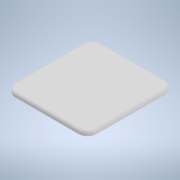
# Autodesk Inventor part: micro lipo lid
Saved by Autodesk Inventor 2020 (Build 240168000, 168)
## iProperties
Created: 2020-08-31
Part Number: micro lipo lid
Material: Generic
Document SubType Name: Modeling
Designer: mulve
Density: 1 g/cm^3
Appearance: Default
Author: mulve
Autodesk Inventor part; units mm, degrees
ref_plane "YZ Plane" through (0, 0, 0) normal (1, 0, 0) x (0, 1, 0)
ref_plane "XZ Plane" through (0, 0, 0) normal (0, 1, 0) x (-1, 0, 0)
ref_plane "XY Plane" through (0, 0, 0) normal (0, 0, 1) x (1, 0, 0)
sketch "Sketch1" plane through (0, 0, 0) normal (0, 1, 0) x (-1, 0, 0)
  line L0 (0, 0) -> (22.86, 0)
  line L1 (22.86, 0) -> (22.86, -24.13)
  line L2 (22.86, -24.13) -> (0, -24.13)
  line L3 (0, -24.13) -> (0, 0)
  dimension "d0" = 24.13
  dimension "d1" = 22.86
  constraints: 8 end point, 2 parallel, 1 horizontal, 1 perpendicular
  measures "d0" distance of L0.end L1.end
  measures "d1" distance of L1.end L2.end
extrude "Extrusion1" add sketch "Sketch1" along normal blind 2
sketch "Sketch2" plane through (0, 0, 0) normal (0, -1, 0) x (1, 0, 0)
  line L0 (-1.27, -1.27) -> (-21.59, -1.27)
  line L1 (-21.59, -1.27) -> (-21.59, -22.86)
  line L2 (-21.59, -22.86) -> (-1.27, -22.86)
  line L3 (-1.27, -22.86) -> (-1.27, -1.27)
  line L4 (-22.86, 0) -> (0, 0) projected
  line L5 (0, -24.13) -> (-22.86, -24.13) projected
  line L6 (0, 0) -> (0, -24.13) projected
  line L7 (-22.86, -24.13) -> (-22.86, 0) projected
  line L8 (0, 0) -> (0, -24.13) projected
  line L9 (0, 0) -> (-22.86, 0)
  line L10 (-22.86, 0) -> (-22.86, -24.13)
  line L11 (-22.86, -24.13) -> (0, -24.13)
  line L12 (0, -24.13) -> (0, 0)
  dimension "d4" = 20.32
  dimension "d5" = 21.59
  dimension "d6" = 1.27
  dimension "d7" = 1.27
  dimension "d8" = 1.27
  dimension "d9" = 1.27
  constraints: 16 end point, 4 parallel, 2 horizontal, 2 perpendicular
  measures "d4" distance of L1.end L2.end
  measures "d5" distance of L2.end L0.start
  measures "d6" distance between parallel lines of L4 L0
  measures "d7" distance between parallel lines of L5 L2
  measures "d8" distance between parallel lines of L6 L3
  measures "d9" distance between parallel lines of L7 L1
extrude "Extrusion2" cut sketch "Sketch2" against normal blind 0.8
fillet "Fillet1" radius 2.54 8 edges at (0, 1.4, 0) (0, 1.4, -24.13) (-22.86, 1.4, -24.13) (-22.86, 1.4, 0) (-21.59, 0.4, -1.27) (-1.27, 0.4, -1.27) (-1.27, 0.4, -22.86) (-21.59, 0.4, -22.86)
fillet "Fillet2" radius 0.635 8 edges at (-22.1161, 2, -0.7439) (-11.43, 2, 0) (-0.7439, 2, -0.7439) (0, 2, -12.065) (-0.7439, 2, -23.3861) (-11.43, 2, -24.13) (-22.1161, 2, -23.3861) (-22.86, 2, -12.065)
equation "\"d6\" = d7"
equation "\"d8\" = d9"
body "Solid1"
